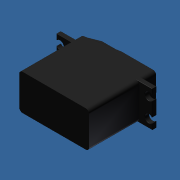
# Autodesk Inventor part: carcaza servo power modificado
Saved by Autodesk Inventor 2014 (Build 180170000, 170)
## iProperties
Created: 2010-09-11
Part Number: carcaza servo power modificado
Document SubType Name: Modeling
Designer: LEFO
Density: 1 g/cm^3
Material: Generic
Appearance: Glossy - Black
Author: LEFO
Autodesk Inventor part; units mm, degrees
ref_plane "YZ Plane" through (0, 0, 0) normal (1, 0, 0) x (0, 1, 0)
ref_plane "XZ Plane" through (0, 0, 0) normal (0, 1, 0) x (-1, 0, 0)
ref_plane "XY Plane" through (0, 0, 0) normal (0, 0, 1) x (1, 0, 0)
sketch "Sketch1" plane through (0, 0, 0) normal (0, 0, 1) x (1, 0, 0)
  line L0 (-13.8273, 26.0318) -> (26.6727, 26.0318)
  line L1 (26.6727, 26.0318) -> (26.6727, -13.4682)
  line L2 (26.6727, -13.4682) -> (-13.8273, -13.4682)
  line L3 (-13.8273, -13.4682) -> (-13.8273, 26.0318)
  line L4 (10.1727, 28.0318) -> (23.1727, 28.0318)
  line L5 (23.1727, 28.0318) -> (23.1727, 26.0318)
  line L6 (23.1727, 26.0318) -> (10.1727, 26.0318)
  line L7 (10.1727, 26.0318) -> (10.1727, 28.0318)
  line L8 (26.6727, 18.0318) -> (34.1727, 18.0318)
  line L9 (34.1727, 18.0318) -> (34.1727, 15.5318)
  line L10 (34.1727, 15.5318) -> (26.6727, 15.5318)
  line L11 (26.6727, 15.5318) -> (26.6727, 18.0318)
  line L12 (6.4227, -13.4682) -> (6.4227, 46.607) construction
  line L13 (-13.8273, 18.0318) -> (-21.3273, 18.0318)
  line L14 (-21.3273, 18.0318) -> (-21.3273, 15.5318)
  line L15 (-21.3273, 15.5318) -> (-13.8273, 15.5318)
  line L16 (-13.8273, 15.5318) -> (-13.8273, 18.0318)
  dimension "d2" = 40.5
  dimension "d3" = 39.5
  dimension "d4" = 2
  dimension "d5" = 13
  dimension "d6" = 3.5
  dimension "d7" = 7.5
  dimension "d8" = 2.5
  dimension "d9" = 8
  dimension "d11" = 28.5751
  constraints: 34 end point, 7 parallel, 4 symmetric about line, 3 horizontal, 3 perpendicular, 2 collinear, 1 midpoint
  measures "d2" distance of L1.end L2.end
  measures "d3" distance of L0.end L1.end
  measures "d4" distance of L4.end L5.end
  measures "d5" distance of L4.start L4.end
  measures "d6" distance between parallel lines of L1 L5
  measures "d7" distance of L9.end L10.end
  measures "d8" distance of L8.end L9.end
  measures "d9" distance between parallel lines of L8 L0
  measures "d11" distance from line of L12.end L8
extrude "Extrusion1" add sketch "Sketch1" along normal blind 20.7
sketch "Sketch2" plane through (10.1727, 28.0318, 0) normal (0, 1, 0) x (1, 0, 0)
  line L0 (0, -20.7) -> (13, -20.7) projected
  line L1 (13, 0) -> (13, -20.7) projected
  line L2 (0, 0) -> (13, 0) projected
  line L3 (0, 0) -> (0, -20.7) projected
  circle A0 centre (6.5, -10.35) radius 6.5
  point P0 (6.5, 0)
  point P1 (0, -10.35)
  dimension "d14" = 13
  constraints: 2 midpoint, 1 centre point, 1 horizontal alignment, 1 vertical alignment
  measures "d14" diameter of A0
extrude "Extrusion2" cut sketch "Sketch2" against normal up to surface (2 mm away) contours L3 A0 L1 L0 | L3 L2 L1 A0
sketch "Sketch3" plane through (16.6727, 28.0318, 10.35) normal (0, 1, 0) x (1, 0, 0)
  circle A0 centre (0, 0) radius 6.5 projected
  circle A1 centre (0, 0) radius 4.5
  dimension "d17" = 9
  constraints: 1 centre point, 1 coincident
  measures "d17" diameter of A1
extrude "Extrusion3" cut sketch "Sketch3" against normal blind 0.5
sketch "Sketch4" plane through (-13.8273, 26.0318, 0) normal (0, 1, 0) x (1, 0, 0)
  line L0 (0, 0) -> (40.5, 0) projected
  line L1 (0, 0) -> (0, -20.7) projected
  line L2 (0, -20.7) -> (40.5, -20.7) projected
  line L3 (40.5, 0) -> (40.5, -20.7) projected
  line L4 (1, -1) -> (39.5, -1)
  line L5 (39.5, -1) -> (39.5, -19.7)
  line L6 (39.5, -19.7) -> (1, -19.7)
  line L7 (1, -19.7) -> (1, -1)
  dimension "d20" = 1
  dimension "d21" = 1
  dimension "d22" = 1
  dimension "d23" = 1
  constraints: 8 end point, 2 parallel, 1 horizontal, 1 perpendicular
  measures "d20" distance between parallel lines of L4 L0
  measures "d21" distance between parallel lines of L1 L7
  measures "d22" distance between parallel lines of L3 L5
  measures "d23" distance between parallel lines of L2 L6
extrude "Extrusion4" cut sketch "Sketch4" against normal blind 0.5
sketch "Sketch5" plane through (0, 0, 20.7) normal (0, 0, 1) x (1, 0, 0)
  line L0 (26.6727, 25.5318) -> (-13.8273, 25.5318) projected
  line L1 (26.6727, 25.5318) -> (6.6727, 25.5318)
  line L2 (-13.8273, 25.5318) -> (-13.8273, 22.0318)
  line L3 (-13.8273, 22.0318) -> (6.6727, 25.5318)
  line L4 (-12.2624, 22.299) -> (-12.2624, 23.299)
  line L5 (-12.8273, 26.0318) -> (25.6727, 26.0318) projected
  line L6 (-12.8273, 26.0318) -> (-12.8273, 25.5318) projected
  line L7 (25.6727, 26.0318) -> (25.6727, 25.5318) projected
  line L8 (-5.3273, 26.0318) -> (-5.3273, 30.9826)
  line L9 (-12.2624, 23.299) -> (-5.3273, 26.0318)
  line L10 (-5.3273, 26.0318) -> (-13.8273, 26.0318)
  line L11 (-13.8273, 26.0318) -> (-13.8273, 25.5318)
  line L12 (-6.5962, 25.5318) -> (6.6727, 25.5318)
  dimension "d26" = 20
  dimension "d28" = 3.5
  dimension "d29" = 1
  dimension "d30" = 12
  dimension "d36" = 158.493
  constraints: 18 end point, 6 point on line, 2 collinear, 2 perpendicular, 1 parallel
  measures "d26" distance of L0.start L1.end
  measures "d28" distance of L0.end L2.end
  measures "d29" distance of L4.start L4.end
  measures "d30" distance from line of L1.end L8
  measures "d36" angle of L10 L9
extrude "Extrusion5" cut sketch "Sketch5" against normal up to surface (20.7 mm away) contours L9 L4 L3 L2 L0 | L0 L6 L5 L9
extrude "Extrusion6" cut sketch "Sketch5" against normal blind 1 contours L3 L4 L9 L0
sketch "Sketch6" plane through (0, 0, 0) normal (0, 0, -1) x (-1, 0, 0)
  line L0 (12.2624, 22.299) -> (12.2624, 23.299) projected
  line L1 (12.2624, 23.299) -> (6.5962, 25.5318) projected
  line L2 (6.5962, 25.5318) -> (-26.6727, 25.5318) projected
  line L3 (12.2624, 22.299) -> (-6.6727, 25.5318) projected
  line L4 (-6.6727, 25.5318) -> (6.5962, 25.5318)
  line L5 (12.2624, 23.299) -> (12.2624, 22.299)
  line L6 (-6.6727, 25.5318) -> (12.2624, 22.299)
  line L7 (6.5962, 25.5318) -> (12.2624, 23.299)
  constraints: 8 end point, 3 collinear, 1 perpendicular
extrude "Extrusion7" cut sketch "Sketch6" against normal blind 1
sketch "Sketch7" plane through (26.6727, 18.0318, 0) normal (0, 1, 0) x (1, 0, 0)
  line L0 (7.5, 0) -> (7.5, -20.7) projected
  line L1 (0, 0) -> (7.5, 0) projected
  line L2 (0, 0) -> (0, -20.7) projected
  circle A0 centre (5.5, -4.75) radius 2.25
  line L3 (7.5, -10.35) -> (-4.0351, -10.35) construction
  circle A1 centre (5.5, -15.95) radius 2.25
  line L4 (-20, 0) -> (0, 0) projected
  line L5 (-40.5, 0) -> (-20, 0) projected
  dimension "d43" = 4.5
  dimension "d44" = 2
  dimension "d45" = 4.75
  constraints: 2 centre point, 2 end point, 1 midpoint, 1 perpendicular, 1 symmetric about line, 1 other
  measures "d43" diameter of A0
  measures "d44" distance from line of L0 A0.centre
  measures "d45" distance from line of L1 A0.centre
extrude "Extrusion8" cut sketch "Sketch7" against normal up to surface (2.5 mm away)
ref_plane "Work Plane2" through (6.4227, -13.4682, 0) normal (-1, 0, 0) x (0, 0, 1)
mirror "Mirror1" about plane through (6.4227, -13.4682, 0) normal (-1, 0, 0) of "Extrusion8"
ref_plane "Work Plane4" through (0, 0, 10.35) normal (0, 0, 1) x (1, 0, 0)
sketch "Sketch8" plane through (0, 0, 10.35) normal (0, 0, 1) x (1, 0, 0)
  line L0 (-13.8273, 18.0318) -> (-13.8273, 22.0318) projected
  line L1 (-21.3273, 18.0318) -> (-13.8273, 18.0318) projected
  line L2 (26.6727, 25.5318) -> (26.6727, 18.0318) projected
  line L3 (26.6727, 18.0318) -> (34.1727, 18.0318) projected
  line L4 (6.6727, 25.5318) -> (-13.8273, 22.0318) projected
  line L5 (-13.8273, 18.0318) -> (-13.8273, 22.0318) projected
  line L6 (-21.3273, 18.0318) -> (-13.8273, 18.0318) projected
  line L7 (-21.3273, 15.5318) -> (-21.3273, 18.0318) projected
  line L8 (-13.8273, 15.5318) -> (-21.3273, 15.5318) projected
  line L9 (-13.8273, -13.4682) -> (-13.8273, 15.5318) projected
  line L10 (26.6727, -13.4682) -> (-13.8273, -13.4682) projected
  line L11 (26.6727, 15.5318) -> (26.6727, -13.4682) projected
  line L12 (34.1727, 15.5318) -> (26.6727, 15.5318) projected
  line L13 (34.1727, 18.0318) -> (34.1727, 15.5318) projected
  line L14 (26.6727, 18.0318) -> (34.1727, 18.0318) projected
  line L15 (26.6727, 25.5318) -> (26.6727, 18.0318) projected
  line L16 (26.6727, 25.5318) -> (6.6727, 25.5318) projected
  line L17 (-18.8273, 18.0318) -> (-13.8273, 20.7318)
  line L18 (-13.8273, 20.7318) -> (-13.8273, 18.0318)
  line L19 (-13.8273, 18.0318) -> (-18.8273, 18.0318)
  line L20 (6.4227, -13.4682) -> (6.4227, 33.9589) construction
  line L21 (31.6727, 18.0318) -> (26.6727, 20.7318)
  line L22 (26.6727, 20.7318) -> (26.6727, 18.0318)
  line L23 (26.6727, 18.0318) -> (31.6727, 18.0318)
  dimension "d53" = 2.7
  dimension "d54" = 5
  constraints: 14 end point, 3 symmetric about line, 2 perpendicular, 2 point on line, 1 collinear, 1 midpoint
  measures "d53" distance of L17.end L5.start
  measures "d54" distance of L5.start L17.start
extrude "Extrusion9" add sketch "Sketch8" along normal mid plane 2 contours L1 L17 L0 | L21 L3 L2
chamfer "Chamfer1" distance 0.3 angle 45 1 edges at (12.1727, 28.0318, 10.35)
chamfer "Chamfer2" distance 1 angle 45 1 edges at (10.1727, 27.5318, 10.35)
fillet "Fillet1" radius 2 8 edges at (-13.8273, 1.0318, 20.7) (-13.8273, 20.0318, 20.7) (-13.8273, 20.0318, 0) (-13.8273, 1.0318, 0) (26.6727, 21.7818, 20.7) (26.6727, 1.0318, 20.7) (26.6727, 21.7818, 0) (26.6727, 1.0318, 0)
fillet "Fillet2" radius 0.3 12 edges at (-12.2624, 23.299, 10.35) (-13.8273, 22.0318, 10.35) (-13.2416, 22.1318, 0.5858) (-2.5773, 23.9525, 0) (-13.2416, 22.1318, 20.1142) (-2.5773, 23.9525, 20.7) (15.6727, 25.5318, 20.7) (26.0869, 25.5318, 20.1142) (26.6727, 25.5318, 10.35) (26.0869, 25.5318, 0.5858) (15.6727, 25.5318, 0) (-5.3273, 26.0318, 10.35)
fillet "Fillet3" radius 2 2 edges at (25.6727, 25.7818, 1) (25.6727, 25.7818, 19.7)
fillet "Fillet3" radius 0.3 11 edges at (10.2011, 26.0318, 1) (-5.3263, 26.0265, 1) (-8.7264, 24.6924, 1) (-12.2104, 23.2636, 1) (-12.2624, 22.6969, 1) (10.2011, 26.0318, 19.7) (-5.3263, 26.0265, 19.7) (-8.7264, 24.6924, 19.7) (-12.2104, 23.2636, 19.7) (-12.2624, 22.6969, 19.7) (25.6727, 26.0318, 10.35)
fillet "Fillet4" radius 0.2 44 edges at (-21.3273, 16.7818, 3.7192) (-21.3273, 16.7818, 5.7808) (-21.3273, 16.7818, 14.9192) (-21.3273, 16.7818, 16.9808) (34.1727, 16.7818, 3.7192) (34.1727, 16.7818, 14.9192) (34.1727, 16.7818, 5.7808) (34.1727, 16.7818, 16.9808) (-12.8273, 18.0318, 0) (-17.5773, 18.0318, 0) (-21.3273, 18.0318, 1.8596) (-21.3273, 16.7818, 0) (-21.3273, 15.5318, 1.8596) (-17.0773, 18.0318, 4.75) (-17.0773, 15.5318, 4.75) (-17.0773, 18.0318, 15.95) (-17.0773, 15.5318, 15.95) (-12.8273, 18.0318, 20.7) (-17.5773, 18.0318, 20.7) (-17.5773, 15.5318, 20.7) (-12.8273, 15.5318, 20.7) (-21.3273, 16.7818, 20.7) (-21.3273, 15.5318, 18.8404) (-21.3273, 18.0318, 18.8404) (-21.3273, 18.0318, 10.35) (-21.3273, 15.5318, 10.35) (29.9227, 18.0318, 4.75) (29.9227, 15.5318, 4.75) (29.9227, 18.0318, 15.95) (29.9227, 15.5318, 15.95) (34.1727, 18.0318, 10.35) (34.1727, 15.5318, 10.35) (34.1727, 15.5318, 1.8596) (34.1727, 18.0318, 1.8596) (25.6727, 18.0318, 0) (30.4227, 18.0318, 0) (30.4227, 15.5318, 0) (25.6727, 15.5318, 0) (34.1727, 18.0318, 18.8404) (34.1727, 15.5318, 18.8404) (30.4227, 15.5318, 20.7) (25.6727, 15.5318, 20.7) (25.6727, 18.0318, 20.7) (30.4227, 18.0318, 20.7)
hole "Hole1" at (16.6727, 28.0318, 10.35) direction (0, -1, 0) diameter 5.5 depth 8
sketch "Sketch10" plane through (0, 0, 20.7) normal (0, 0, 1) x (1, 0, 0)
  line L0 (-13.8273, 18.0318) -> (-18.8273, 18.0318) projected
  line L1 (-13.8273, 20.7318) -> (-13.8273, 18.0318) projected
  line L2 (-18.8273, 18.0318) -> (-13.8273, 20.7318) projected
  line L3 (31.6727, 18.0318) -> (26.6727, 18.0318) projected
  line L4 (26.6727, 20.7318) -> (31.6727, 18.0318) projected
  line L5 (26.6727, 18.0318) -> (26.6727, 20.7318) projected
  point P0 (0, 0)
extrude "Extrusion10" cut sketch "Sketch10" against normal up to next
equation "\"espesor\" = 20.7"
equation "\"d52\" = -0.5 * espesor"
body "Solid1"
